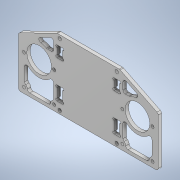
# Autodesk Inventor part: Trunk_horizontal_frame_01
Saved by Autodesk Inventor 2020.4 (Build 244396000, 396)
## iProperties
Created: 2021-09-21
Part Number: Trunk_horizontal_frame_01
Material: アルミニウム 2014-T4
Document SubType Name: Modeling
Designer: Masato
Density: 2.8 g/cm^3
Appearance: 滑らか - 淡い灰色
Author: Masato
Autodesk Inventor part; units mm, degrees
ref_plane "YZ Plane" through (0, 0, 0) normal (1, 0, 0) x (0, 1, 0)
ref_plane "XZ Plane" through (0, 0, 0) normal (0, 1, 0) x (-1, 0, 0)
ref_plane "XY Plane" through (0, 0, 0) normal (0, 0, 1) x (1, 0, 0)
sketch "スケッチ1" plane through (0, 0, 0) normal (0, 0, 1) x (1, 0, 0)
  line L0 (-62.5, 30.75) -> (62.5, 30.75)
  line L1 (62.5, 30.75) -> (62.5, -30.75)
  line L2 (62.5, -30.75) -> (-62.5, -30.75)
  line L3 (-62.5, -30.75) -> (-62.5, 30.75)
  line L4 (-62.5, 30.75) -> (62.5, -30.75) construction
  line L5 (62.5, 30.75) -> (-62.5, -30.75) construction
  line L6 (-62.5, 2.25) -> (62.5, 2.25) construction
  circle A0 centre (-44, 2.25) radius 18.5 construction
  line L7 (-62.5, 0) -> (62.5, 0) construction
  line L8 (0, 30.75) -> (0, -30.75) construction
  circle A1 centre (-44, 2.25) radius 10.5 construction
  line L9 (-57.5, 1.25) -> (-30.5, 1.25) construction
  line L10 (-30.5, 1.25) -> (-30.5, -25.75) construction
  line L11 (-30.5, -25.75) -> (-57.5, -25.75) construction
  line L12 (-57.5, -25.75) -> (-57.5, 1.25) construction
  line L13 (-44, 1.25) -> (-44, -25.75) construction
  line L14 (-57.5, -12.25) -> (-30.5, -12.25) construction
  circle A2 centre (-57.5, 1.25) radius 1.35
  circle A3 centre (-57.5, -25.75) radius 1.35
  circle A4 centre (-30.5, 1.25) radius 1.35
  circle A5 centre (-30.5, -25.75) radius 1.35
  line L15 (-28, 21.75) -> (-23, 21.75) construction
  line L16 (-23, 21.75) -> (-23, 11.75) construction
  line L17 (-23, 11.75) -> (-28, 11.75) construction
  line L18 (-28, 11.75) -> (-28, 21.75) construction
  line L19 (-28, 21.75) -> (-23, 11.75) construction
  line L20 (-23, 21.75) -> (-28, 11.75) construction
  line L21 (-28.01, 21.76) -> (-22.99, 21.76)
  line L22 (-22.99, 21.76) -> (-22.99, 11.74)
  line L23 (-22.99, 11.74) -> (-28.01, 11.74)
  line L24 (-28.01, 11.74) -> (-28.01, 21.76)
  line L25 (-28.01, 21.76) -> (-22.99, 11.74) construction
  line L26 (-22.99, 21.76) -> (-28.01, 11.74) construction
  line L27 (-28.01, 16.75) -> (-22.99, 16.75) construction
  line L28 (-25.5, 21.76) -> (-25.5, 11.74) construction
  arc A6 (-28.01, 21.76) -> (-28.01, 19.66) centre (-28.01, 20.71) ccw
  arc A7 (-22.99, 19.66) -> (-22.99, 21.76) centre (-22.99, 20.71) ccw
  arc A8 (-28.01, 13.84) -> (-28.01, 11.74) centre (-28.01, 12.79) ccw
  arc A9 (-22.99, 11.74) -> (-22.99, 13.84) centre (-22.99, 12.79) ccw
  circle A10 centre (-25.5, 27.75) radius 1.55
  line L29 (-28, -9.25) -> (-23, -9.25) construction
  line L30 (-23, -9.25) -> (-23, -21.75) construction
  line L31 (-23, -21.75) -> (-28, -21.75) construction
  line L32 (-28, -21.75) -> (-28, -9.25) construction
  line L33 (-28, -9.25) -> (-23, -21.75) construction
  line L34 (-23, -9.25) -> (-28, -21.75) construction
  line L35 (-28.01, -9.24) -> (-22.99, -9.24)
  line L36 (-22.99, -9.24) -> (-22.99, -21.76)
  line L37 (-22.99, -21.76) -> (-28.01, -21.76)
  line L38 (-28.01, -21.76) -> (-28.01, -9.24)
  line L39 (-28.01, -9.24) -> (-22.99, -21.76) construction
  line L40 (-22.99, -9.24) -> (-28.01, -21.76) construction
  line L41 (-28.01, -15.5) -> (-22.99, -15.5) construction
  line L42 (-25.5, -9.24) -> (-25.5, -21.76) construction
  arc A11 (-28.01, -9.24) -> (-28.01, -11.34) centre (-28.01, -10.29) ccw
  arc A12 (-22.99, -11.34) -> (-22.99, -9.24) centre (-22.99, -10.29) ccw
  arc A13 (-22.99, -21.76) -> (-22.99, -19.66) centre (-22.99, -20.71) ccw
  arc A14 (-28.01, -19.66) -> (-28.01, -21.76) centre (-28.01, -20.71) ccw
  circle A15 centre (-25.5, -27.75) radius 1.55
  circle A16 centre (-44, 2.25) radius 11
  arc A17 (-54.9991, 2.3936) -> (-54.8579, 0.4874) centre (-57.5, 1.25) ccw
  arc A18 (-33.1421, 0.4874) -> (-33.0009, 2.3936) centre (-30.5, 1.25) ccw
  line L43 (62.5, 30.75) -> (-62.5, -30.75) construction
  line L44 (-62.5, 30.75) -> (62.5, -30.75) construction
  line L45 (62.5, 2.25) -> (-62.5, 2.25) construction
  circle A19 centre (44, 2.25) radius 18.5 construction
  line L46 (62.5, 0) -> (-62.5, 0) construction
  circle A20 centre (44, 2.25) radius 10.5 construction
  line L47 (57.5, 1.25) -> (30.5, 1.25) construction
  line L48 (30.5, 1.25) -> (30.5, -25.75) construction
  line L49 (30.5, -25.75) -> (57.5, -25.75) construction
  line L50 (57.5, -25.75) -> (57.5, 1.25) construction
  line L51 (44, 1.25) -> (44, -25.75) construction
  line L52 (57.5, -12.25) -> (30.5, -12.25) construction
  circle A21 centre (57.5, 1.25) radius 1.35
  circle A22 centre (57.5, -25.75) radius 1.35
  circle A23 centre (30.5, 1.25) radius 1.35
  circle A24 centre (30.5, -25.75) radius 1.35
  line L53 (28, 21.75) -> (23, 21.75) construction
  line L54 (23, 21.75) -> (23, 11.75) construction
  line L55 (23, 11.75) -> (28, 11.75) construction
  line L56 (28, 11.75) -> (28, 21.75) construction
  line L57 (28, 21.75) -> (23, 11.75) construction
  line L58 (23, 21.75) -> (28, 11.75) construction
  line L59 (28.01, 21.76) -> (22.99, 21.76)
  line L60 (22.99, 21.76) -> (22.99, 11.74)
  line L61 (22.99, 11.74) -> (28.01, 11.74)
  line L62 (28.01, 11.74) -> (28.01, 21.76)
  line L63 (28.01, 21.76) -> (22.99, 11.74) construction
  line L64 (22.99, 21.76) -> (28.01, 11.74) construction
  line L65 (28.01, 16.75) -> (22.99, 16.75) construction
  line L66 (25.5, 21.76) -> (25.5, 11.74) construction
  arc A25 (28.01, 19.66) -> (28.01, 21.76) centre (28.01, 20.71) ccw
  arc A26 (22.99, 21.76) -> (22.99, 19.66) centre (22.99, 20.71) ccw
  arc A27 (22.99, 13.84) -> (22.99, 11.74) centre (22.99, 12.79) ccw
  arc A28 (28.01, 11.74) -> (28.01, 13.84) centre (28.01, 12.79) ccw
  circle A29 centre (25.5, 27.75) radius 1.55
  arc A30 (28.01, -21.76) -> (28.01, -19.66) centre (28.01, -20.71) ccw
  line L67 (23, -21.75) -> (28, -21.75) construction
  line L68 (22.99, -21.76) -> (28.01, -21.76)
  arc A31 (22.99, -19.66) -> (22.99, -21.76) centre (22.99, -20.71) ccw
  line L69 (28, -21.75) -> (28, -9.25) construction
  line L70 (28.01, -21.76) -> (28.01, -9.24)
  line L71 (28.01, -15.5) -> (22.99, -15.5) construction
  line L72 (25.5, -9.24) -> (25.5, -21.76) construction
  line L73 (28, -9.25) -> (23, -21.75) construction
  line L74 (23, -9.25) -> (28, -21.75) construction
  line L75 (28.01, -9.24) -> (22.99, -21.76) construction
  line L76 (22.99, -9.24) -> (28.01, -21.76) construction
  line L77 (23, -9.25) -> (23, -21.75) construction
  line L78 (22.99, -9.24) -> (22.99, -21.76)
  circle A32 centre (25.5, -27.75) radius 1.55
  arc A33 (22.99, -9.24) -> (22.99, -11.34) centre (22.99, -10.29) ccw
  line L79 (28, -9.25) -> (23, -9.25) construction
  line L80 (28.01, -9.24) -> (22.99, -9.24)
  arc A34 (28.01, -11.34) -> (28.01, -9.24) centre (28.01, -10.29) ccw
  circle A35 centre (44, 2.25) radius 11
  arc A36 (54.8579, 0.4874) -> (54.9991, 2.3936) centre (57.5, 1.25) ccw
  arc A37 (33.0009, 2.3936) -> (33.1421, 0.4874) centre (30.5, 1.25) ccw
  arc A38 (-44, -11.75) -> (-31.01, -2.9711) centre (-44, 2.25) ccw
  arc A39 (-55.2639, -27.75) -> (-56.99, -22.7937) centre (-57.5, -25.75) ccw
  line L81 (-56.99, -22.7937) -> (-56.99, -2.9711)
  line L82 (-55.2639, -27.75) -> (-32.7361, -27.75)
  arc A40 (-31.01, -22.7937) -> (-32.7361, -27.75) centre (-30.5, -25.75) ccw
  line L83 (-31.01, -22.7937) -> (-31.01, -2.9711)
  arc A41 (-56.99, -2.9711) -> (-44, -11.75) centre (-44, 2.25) ccw
  arc A42 (31.01, -2.9711) -> (44, -11.75) centre (44, 2.25) ccw
  arc A43 (56.99, -22.7937) -> (55.2639, -27.75) centre (57.5, -25.75) ccw
  line L84 (56.99, -22.7937) -> (56.99, -2.9711)
  line L85 (55.2639, -27.75) -> (32.7361, -27.75)
  arc A44 (32.7361, -27.75) -> (31.01, -22.7937) centre (30.5, -25.75) ccw
  line L86 (31.01, -22.7937) -> (31.01, -2.9711)
  arc A45 (44, -11.75) -> (56.99, -2.9711) centre (44, 2.25) ccw
  line L87 (-60, 14.25) -> (-28, 14.25) construction
  line L88 (-28, 14.25) -> (-28, -28.75) construction
  line L89 (-28, -28.75) -> (-60, -28.75) construction
  line L90 (-60, -28.75) -> (-60, 14.25) construction
  line L91 (-60, 14.25) -> (-28, -28.75) construction
  line L92 (-28, 14.25) -> (-60, -28.75) construction
  arc A46 (-54.583, 14.25) -> (-60, 2.25) centre (-44, 2.25) ccw construction
  arc A47 (-28, 2.25) -> (-33.417, 14.25) centre (-44, 2.25) ccw construction
  line L93 (-28, 30.75) -> (-62.5, 13.7615)
  line L94 (28, 30.75) -> (62.5, 13.7615)
  line L95 (-31.01, 25.9238) -> (-43.143, 19.9493)
  arc A48 (-56.99, -2.9711) -> (-56.1, -4.792) centre (-44, 2.25) ccw
  arc A49 (-43.143, 19.9493) -> (-42.477, 16.1669) centre (-42.2595, 18.155) ccw
  line L96 (-31.01, 14.25) -> (-36.7889, 14.25)
  arc A50 (-36.7889, 14.25) -> (-42.477, 16.1669) centre (-44, 2.25) ccw
  line L97 (-31.01, 14.25) -> (-31.01, 25.9238)
  line L98 (31.01, 25.9238) -> (43.143, 19.9493)
  arc A51 (42.477, 16.1669) -> (43.143, 19.9493) centre (42.2595, 18.155) ccw
  line L99 (31.01, 14.25) -> (36.7889, 14.25)
  arc A52 (42.477, 16.1669) -> (36.7889, 14.25) centre (44, 2.25) ccw
  line L100 (31.01, 14.25) -> (31.01, 25.9238)
  point P0 (0, 0)
  point P1 (-25.5, 16.75)
  point P2 (-25.5, -15.5)
  point P3 (25.5, 16.75)
  point P4 (25.5, -15.5)
  point P5 (28.01, -19.66)
  point P6 (22.99, -11.34)
  point P7 (22.99, 19.66)
  point P8 (28.01, 13.84)
  point P9 (-28.01, -19.66)
  point P10 (-22.99, -19.66)
  point P11 (-22.99, 13.84)
  point P12 (-44, -7.25)
  dimension "d2" = 37
  dimension "d3" = 21
  dimension "d4" = 27
  dimension "d5" = 2.7
  dimension "d6" = 1
  dimension "d7" = 27
  dimension "d8" = 5
  dimension "d9" = 10
  dimension "d10" = 0.01
  dimension "d11" = 0.01
  dimension "d12" = 1.05
  dimension "d13" = 3.1
  dimension "d14" = 5
  dimension "d15" = 12.5
  dimension "d16" = 0.01
  dimension "d17" = 0.01
  dimension "d18" = 1.05
  dimension "d19" = 3.1
  dimension "d20" = 6
  dimension "d21" = 6
  dimension "d22" = 44
  dimension "d23" = 16
  dimension "d24" = 3
  dimension "d25" = 3
  dimension "d26" = 28.5
  dimension "d28" = 33
  dimension "d29" = 0.5
  dimension "d31" = 2.75
  dimension "d32" = 11.5
  dimension "d33" = 10.5
  dimension "d34" = 10.5
  dimension "d35" = 18.5
  dimension "d36" = 125
  dimension "d39" = 3
  dimension "d40" = 3
  dimension "d41" = 3
  dimension "d42" = 3
  dimension "d45" = 32
  dimension "d46" = 43
  dimension "d47" = 9.5
  dimension "d48" = 2
  dimension "d49" = 2.5
  dimension "d50" = 16
  dimension "d52" = 3
  dimension "d54" = 2
  dimension "d55" = 3
  constraints: 202 end point, 115 symmetric about line, 75 point on circle, 53 centre point, 36 midpoint, 28 point on line, 15 parallel, 12 coincident, 8 horizontal, 8 perpendicular, 3 tangent, 3 vertical, 1 collinear, 37 other
  measures "d2" diameter of A0
  measures "d3" diameter of A1
  measures "d4" distance of L10.end L11.end
  measures "d5" diameter of A2
  measures "d6" distance of L13.start A0.centre
  measures "d7" distance of L10.end L9.end
  measures "d8" distance of L16.end L17.end
  measures "d9" distance of L15.end L16.end
  measures "d10" distance between parallel lines of L21 L15
  measures "d11" distance between parallel lines of L22 L16
  measures "d12" radius of A6
  measures "d13" diameter of A10
  measures "d14" distance of L31.start L31.end
  measures "d15" distance of L34.start L31.start
  measures "d16" distance between parallel lines of L35 L29
  measures "d17" distance between parallel lines of L36 L30
  measures "d18" radius of A11
  measures "d19" diameter of A15
  measures "d20" vertical distance of L15.end A10.centre
  measures "d21" vertical distance of L31.start A15.centre
  measures "d22" horizontal distance of A0.centre point (0, 0)
  measures "d23" horizontal distance of A0.centre L15.start
  measures "d24" vertical distance of L8.start A10.centre
  measures "d25" distance from line of L2 A15.centre
  measures "d26" vertical distance of A0.centre L8.start
  measures "d28" vertical distance of L2.end A0.centre
  measures "d29" radial gap between concentric circles of A1 A16
  measures "d31" radius of A17
  measures "d32" distance between parallel lines of L29 L6
  measures "d33" vertical distance of L32.end A4.centre
  measures "d34" distance from line of A4.centre L17
  measures "d35" horizontal distance of L0.start A1.centre
  measures "d36" distance of L0.start L0.end
  measures "d39" vertical distance of L2.end L82.start
  measures "d40" radial gap between concentric circles of A38 A16
  measures "d41" radius of A39
  measures "d42" distance from line of L83 A11.centre
  measures "d45" distance of L88.end L89.end
  measures "d46" distance of L87.end L88.end
  measures "d47" distance of point (-44, -7.25) A16.centre
  measures "d48" vertical distance of L2.end L89.end
  measures "d49" horizontal distance of L2.end L89.end
  measures "d50" radius of A46
  measures "d52" distance between parallel lines of L95 L93
  measures "d54" radius of A49
  measures "d55" radial gap between concentric circles of A16 A50
extrude "押し出し1" add sketch "スケッチ1" along normal blind 3 contours L0 L94 L1 L2 L3 L93 | A16 A18 | A16 A17 | A35 A36 | A35 A37
fillet "フィレット1" radius 2 18 edges at (-56.99, -2.9711, 1.5) (-31.01, -2.9711, 1.5) (-56.99, -22.7937, 1.5) (-55.2639, -27.75, 1.5) (-32.7361, -27.75, 1.5) (-31.01, -22.7937, 1.5) (31.01, -22.7937, 1.5) (32.7361, -27.75, 1.5) (31.01, -2.9711, 1.5) (56.99, -2.9711, 1.5) (56.99, -22.7937, 1.5) (55.2639, -27.75, 1.5) (31.01, 25.9238, 1.5) (-31.01, 25.9238, 1.5) (-36.7889, 14.25, 1.5) (-31.01, 14.25, 1.5) (31.01, 14.25, 1.5) (36.7889, 14.25, 1.5)
fillet "フィレット2" radius 2 6 edges at (62.5, -30.75, 1.5) (-62.5, -30.75, 1.5) (-62.5, 13.7615, 1.5) (-28, 30.75, 1.5) (28, 30.75, 1.5) (62.5, 13.7615, 1.5)
equation "\"d11\" = d10"
equation "\"d14\" = d8"
equation "\"d16\" = d10"
equation "\"d17\" = d16"
equation "\"d18\" = d12"
equation "\"d35\" = 0.5 * d2"
